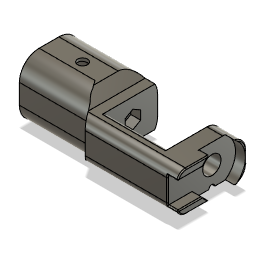
ElbowFork_4 v14 (Autodesk Fusion 360 design; units mm, degrees)
Autodesk Fusion 360 part; units mm, degrees
sketch "Sketch1" plane through (0, 0, 0) normal (0, 1, 0) x (1, 0, 0)
  line L0 (-40, 15) -> (-10, 15)
  line L1 (-10, 15) -> (-10, -15)
  line L2 (-40, -15) -> (-10, -15)
  line L3 (-10, -15) -> (-6.6882, -19.9677)
  line L4 (-5, 0) -> (-5, 15)
  line L5 (27, 0) -> (27, 15)
  line L6 (-5, 0) -> (-5, -10)
  line L7 (-5, -10) -> (27, -10)
  line L8 (27, -10) -> (27, 0)
  line L9 (30, -19.9677) -> (-6.6882, -19.9677)
  line L10 (30, 15) -> (40, 15)
  line L11 (40, 15) -> (40, -19.9677)
  line L12 (40, -19.9677) -> (30, -19.9677)
  line L13 (-10, 15) -> (-5, 15)
  line L14 (27, 15) -> (30, 15)
  line L15 (27, 15) -> (30, 15)
  line L16 (-40, 0) -> (-40, 15)
  line L17 (-40, 0) -> (-40, -15)
  constraint perpendicular L1 L2
  constraint perpendicular L4 L13
  constraint coincident L5.end L13
  constraint parallel L4 L6
  constraint perpendicular L4 L7
  constraint perpendicular L7 L8
  constraint collinear L13 L14
  constraint perpendicular L0 L16
  constraint perpendicular L2 L17
extrude "Extrude1" add sketch "Sketch1" along normal blind 30 makes body 1
sketch "Sketch2" plane through (-40, 0, 0) normal (-1, 0, 0) x (0, 0, 1)
  line L0 (-15, 0) -> (15, 0)
  line L1 (15, 0) -> (15, 30)
  line L2 (15, 30) -> (-15, 30)
  line L3 (-15, 30) -> (-15, 0)
  line L4 (-15, 0) -> (15, 0)
  line L5 (15, 0) -> (15, 30)
  line L6 (15, 30) -> (-15, 30)
  line L7 (-15, 30) -> (-15, 0)
  circle A0 centre (0, 15) radius 13.6
  point P0 (0, 15)
  dimension "d37" = 27.2
  constraint coincident P0 A0.centre
  measures "d37" diameter of A0
extrude "Extrude2" cut sketch "Sketch2" against normal blind 22 contours A0 bodies 1
sketch "Sketch3" plane through (0, 30, 0) normal (0, 1, 0) x (-1, 0, 0)
  line L0 (40, -15) -> (40, 15)
  line L1 (40, 15) -> (10, 15)
  line L2 (10, 15) -> (6.6882, 19.9677)
  line L3 (6.6882, 19.9677) -> (-40, 19.9677)
  line L4 (-40, 19.9677) -> (-40, -15)
  line L5 (-40, -15) -> (-27, -15)
  line L6 (-27, -15) -> (-27, 10)
  line L7 (-27, 10) -> (5, 10)
  line L8 (5, 10) -> (5, -15)
  line L9 (5, -15) -> (40, -15)
  line L10 (10, 15) -> (10, -15)
  constraint coincident L1.end L2.start
  constraint coincident L9 L10.end
  constraint perpendicular L9 L10
extrude "Extrude3" cut sketch "Sketch3" against normal blind 5 contours L2 L3 L4 L5 L6 L7 L8 L9 L10 bodies 1
extrude "Extrude4" cut sketch "Sketch1" along normal blind 5 contours L1 L3 L4 L5 L6 L7 L8 L9 L10 L11 L12 L13 L14 L15 bodies 1
chamfer "Chamfer1" distance 5 angle 45 2 edges at (-10, 30, 0) (-10, 0, 0) on bodies 1
fillet "Fillet1" radius 10 4 edges at (-27.5, 30, -15) (-27.5, 30, 15) (-27.5, 0, -15) (-27.5, 0, 15) on bodies 1
sketch "Sketch4" plane through (40, 0, 0) normal (1, 0, 0) x (0, 0, -1)
  line L0 (-19.9677, 5) -> (15, 5)
  line L1 (15, 5) -> (15, 25)
  line L2 (15, 25) -> (-19.9677, 25)
  line L3 (-19.9677, 25) -> (-19.9677, 5)
  line L4 (2.5, 15) -> (2.5, 5) construction
  circle A0 centre (2.5, 5) radius 1.5
  line L5 (-25, 14.9495) -> (-25, 21.4495)
  line L6 (-25, 14.9495) -> (-25, 8.4495)
  line L7 (-25, 21.4495) -> (-7.6195, 21.4495)
  line L8 (-25, 8.4495) -> (-7.5544, 8.4495)
  arc A1 (-7.5544, 8.4495) -> (-7.6195, 21.4495) centre (2.5, 15) ccw
  circle A2 centre (2.5, 15) radius 4.65
  dimension "d38" = 3
  dimension "d39" = 24
  dimension "d40" = 6.5
  dimension "d41" = 6.5
  dimension "d46" = 9.3
  constraint coincident L0 L4.end
  constraint perpendicular L0 L4
  constraint coincident L4.end A0.centre
  constraint perpendicular L5 L7
  constraint perpendicular L6 L8
  constraint concentric A1 A2
  measures "d38" diameter of A0
  measures "d39" diameter of A1
  measures "d40" distance of L5.start L5.end
  measures "d41" distance of L5.start L6.end
  measures "d46" diameter of A2
extrude "Extrude5" cut sketch "Sketch4" against normal blind 5 contours L0 L2 L3 A0 L7 L8 A1 | A2 bodies 1
extrude "Extrude6" cut sketch "Sketch4" against normal blind 16 contours A2 bodies 1
fillet "Fillet2" radius 2 2 edges at (11, 25, 10) (11, 5, 10) on bodies 1
sketch "Sketch5" plane through (-5, 0, 0) normal (1, 0, 0) x (0, 0, -1)
  arc A0 (13.6603, 5) -> (15, 10) centre (5, 10) ccw
  line L0 (15, 10) -> (15, 20)
  arc A1 (15, 20) -> (13.6603, 25) centre (5, 20) ccw
  line L1 (13.6603, 25) -> (-12, 25)
  arc A2 (-10, 23) -> (-12, 25) centre (-12, 23) ccw
  line L2 (-10, 23) -> (-10, 7)
  arc A3 (-12, 5) -> (-10, 7) centre (-12, 7) ccw
  line L3 (-12, 5) -> (13.6603, 5)
  line L4 (4.45, 11.6225) -> (2.5, 10.4967)
  line L5 (-1.4, 15) -> (-1.4, 17.2517)
  line L6 (0.55, 18.3775) -> (-1.4, 17.2517)
  line L7 (4.45, 18.3775) -> (6.4, 17.2517)
  line L8 (4.45, 18.3775) -> (2.5, 19.5033)
  line L9 (0.55, 18.3775) -> (2.5, 19.5033)
  line L10 (0.55, 11.6225) -> (-1.4, 12.7483)
  line L11 (4.45, 11.6225) -> (6.4, 12.7483)
  line L12 (6.4, 15) -> (6.4, 17.2517)
  line L13 (-1.4, 15) -> (-1.4, 12.7483)
  line L14 (0.55, 11.6225) -> (2.5, 10.4967)
  line L15 (6.4, 15) -> (6.4, 12.7483)
  circle A4 centre (2.5, 15) radius 2.5
  dimension "d36" = 5
  measures "d36" diameter of A4
extrude "Extrude9" cut sketch "Sketch5" against normal blind 5 contours L4 L5 L6 L7 L8 L9 L10 L11 L12 L13 L14 L15 | A4 bodies 1
extrude "Extrude8" cut sketch "Sketch5" against normal blind 15 contours A4 bodies 1
fillet "Fillet3" radius 7 2 edges at (33.5, 25, -15) (33.5, 5, -15) on bodies 1
fillet "Fillet4" radius 4.5 2 edges at (16.6559, 25, 19.9677) (16.6559, 5, 19.9677) on bodies 1
sketch "Sketch6" plane through (0, 30, 0) normal (0, 1, 0) x (-1, 0, 0)
  line L0 (40, 5) -> (16.6667, 5)
  line L1 (16.6667, 5) -> (15, 7.5)
  line L2 (15, 7.5) -> (15, -5)
  line L3 (15, -5) -> (40, -5)
  line L4 (40, -5) -> (40, 5)
  circle A0 centre (28, 0) radius 2.5
  dimension "d33" = 5
  measures "d33" diameter of A0
extrude "Extrude10" cut sketch "Sketch6" against normal blind 58 contours A0 bodies 1
copy_body "Body->Comp1" bodies 1 removing the originals makes body 2 in component "Component"
extrude "Extrude1'" cut 1 faces at (40, 5.54, -2.6771) along direction (-1, 0, 0) blind 9 on bodies 2 bodies 2 in component "Component"
fillet "Fillet1'" radius 0.5 14 edges at (40, 25, 9.8005) (40, 24.0016, 18.2941) (40, 5.9661, 18.2536) (40, 5, 9.8005) (40, 22.4594, -13.3958) (40, 15, -15) (40, 7.5406, -13.3958) (40, 21.4495, 13.7429) (40, 8.4495, 13.6989) (37.5, 21.4495, 19.8664) (37.5, 8.4495, 19.8434) (35, 8.9711, 19.9365) (35, 15, 19.9677) (35, 20.9775, 19.9423) on bodies 2 in component "Component"
move_face "OffsetFaces1" offset 5 1 faces at (-40, 4.1882, 10.0012) on bodies 2 in component "Component"
move_face "OffsetFaces2" offset -1 1 faces at (5.6667, 12.3333, 10) on bodies 2 in component "Component"
component "Component" placed x (1, 0, 0) y (0, 1, 0) z (0, 0, 1) at (0, 0, 0)
